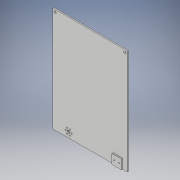
# Autodesk Inventor part: ElectronicsPlate
Saved by Autodesk Inventor 2017 (Build 210142000, 142)
## iProperties
Created: 2018-01-06
Part Number: ElectronicsPlate
Material: Generic
Document SubType Name: Modeling
Designer: User
Density: 1 g/cm^3
Appearance: Default
Author: User
Autodesk Inventor part; units mm, degrees
ref_plane "YZ Plane" through (0, 0, 0) normal (1, 0, 0) x (0, 1, 0)
ref_plane "XZ Plane" through (0, 0, 0) normal (0, 1, 0) x (-1, 0, 0)
ref_plane "XY Plane" through (0, 0, 0) normal (0, 0, 1) x (1, 0, 0)
sketch "Sketch1" plane through (0, 0, 0) normal (0, 0, 1) x (1, 0, 0)
  line L0 (0, 0) -> (199.39, 0)
  line L1 (199.39, 0) -> (199.39, 266.7)
  line L2 (199.39, 266.7) -> (0, 266.7)
  line L3 (0, 266.7) -> (0, 0)
  line L4 (12.1493, 266.7) -> (12.1493, 263.525)
  line L5 (0, 247.1772) -> (3.175, 247.1772)
  line L6 (3.175, 263.525) -> (147.2946, 263.525)
  line L7 (147.2946, 263.525) -> (147.2946, 161.925)
  line L8 (147.2946, 161.925) -> (3.175, 161.925)
  line L9 (3.175, 161.925) -> (3.175, 263.525)
  line L10 (5.8968, 161.925) -> (5.8968, 158.75)
  line L11 (3.175, 158.75) -> (147.2946, 158.75)
  line L12 (147.2946, 158.75) -> (147.2946, 57.15)
  line L13 (147.2946, 57.15) -> (3.175, 57.15)
  line L14 (3.175, 57.15) -> (3.175, 158.75)
  line L15 (147.2946, 247.6224) -> (150.4696, 247.6224)
  line L16 (150.4696, 199.39) -> (186.0296, 199.39)
  line L17 (186.0296, 199.39) -> (186.0296, 107.95)
  line L18 (186.0296, 107.95) -> (150.4696, 107.95)
  line L19 (150.4696, 107.95) -> (150.4696, 199.39)
  dimension "d0" = 199.39
  dimension "d2" = 3.175
  dimension "d3" = 3.175
  dimension "d4" = 144.1196
  dimension "d5" = 101.6
  dimension "d6" = 3.175
  dimension "d7" = 101.6
  dimension "d8" = 3.175
  dimension "d9" = 35.56
  dimension "d10" = 91.44
  dimension "d11" = 107.95
  dimension "d12" = 3.175
  dimension "d13" = 3.175
  constraints: 40 end point, 8 parallel, 7 perpendicular, 5 horizontal, 4 point on line
  measures "d0" distance of L2.end L1.end
  measures "d2" distance of L4.start L4.end
  measures "d3" distance of L5.start L5.end
  measures "d4" distance of L7.end L8.end
  measures "d5" distance of L6.end L7.end
  measures "d6" distance of L10.start L10.end
  measures "d7" distance of L11.end L12.end
  measures "d8" distance of L15.start L15.end
  measures "d9" distance of L17.end L18.end
  measures "d10" distance of L16.end L17.end
  measures "d11" distance between parallel lines of L0 L18
  measures "d12" distance between parallel lines of L2 L6
  measures "d13" distance between parallel lines of L8 L11
sketch "Sketch2" plane through (0, 0, 0) normal (0, 0, 1) x (1, 0, 0)
  line L0 (199.39, 0) -> (0, 0)
  line L1 (0, 0) -> (0, 266.7)
  line L2 (0, 266.7) -> (199.39, 266.7)
  line L3 (199.39, 266.7) -> (199.39, 0)
  point P0 (0, 0)
  constraints: 8 end point, 2 parallel, 1 horizontal, 1 perpendicular
extrude "Extrusion1" add sketch "Sketch2" along normal blind 3.175
sketch "Sketch3" plane through (0, 0, 3.175) normal (0, 0, 1) x (1, 0, 0)
  line L0 (33.6942, 0) -> (33.6942, 14.605)
  line L1 (0, 14.605) -> (42.5196, 14.605)
  line L2 (0, 14.605) -> (42.5196, 14.605) construction
  circle A0 centre (42.5196, 14.605) radius 8.001
  circle A1 centre (42.5196, 14.605) radius 3.4925
  circle A2 centre (34.5186, 14.605) radius 1.5875
  circle A3 centre (38.5191, 7.6759) radius 1.5875
  circle A4 centre (46.5201, 7.6759) radius 1.5875
  circle A5 centre (50.5206, 14.605) radius 1.5875
  circle A6 centre (46.5201, 21.5341) radius 1.5875
  circle A7 centre (38.5191, 21.5341) radius 1.5875
  dimension "d20" = 16.002
  dimension "d16" = 14.605
  dimension "d18" = 42.5196
  dimension "d19" = 0
  dimension "d21" = 6.985
  dimension "d22" = 3.175
  dimension "d27" = 360
  constraints: 7 centre point, 6 end point, 2 coincident, 1 collinear, 1 horizontal, 1 horizontal alignment, 1 point on line, 15 other
  measures "d16" distance of L0.start L0.end
  measures "d18" distance of L1.start L1.end
  measures "d19" distance between parallel lines of L1 L2
  measures "d21" diameter of A1
  measures "d22" diameter of A2
extrude "Extrusion2" cut sketch "Sketch3" against normal blind 6.35 contours A2 L1 L0 | L0 L1 A0 A2 | L1 A2 A0 | A0 L1 A2 | A0 A2 L1 | A3 A0 | A0 A3 | A7 A0 | A0 A7 | A4 A0 | A0 A4 | A6 A0 | A0 A6 | A5 A0 | A0 A5 | A1
sketch "Sketch4" plane through (0, 0, 0) normal (0, 0, -1) x (-1, 0, 0)
  line L0 (-199.39, 0) -> (-199.39, 266.7) projected
  line L1 (-199.39, 15.2095) -> (-180.34, 15.2095)
  line L2 (-199.39, 15.2095) -> (-180.34, 15.2095) construction
  line L3 (0, 0) -> (-199.39, 0) projected
  line L4 (-180.34, 0) -> (-180.34, 12.7)
  line L5 (-180.34, 0) -> (-167.64, 0) construction
  line L6 (-180.34, 12.7) -> (-167.64, 12.7)
  circle A0 centre (-180.34, 12.7) radius 1.7526
  circle A1 centre (-167.64, 12.7) radius 1.7526
  dimension "d29" = 19.05
  dimension "d30" = 0
  dimension "d31" = 12.7
  dimension "d32" = 90
  dimension "d33" = 12.7
  dimension "d34" = 3.5052
  dimension "d35" = 3.5052
  dimension "d48" = 0
  constraints: 10 end point, 3 horizontal, 2 centre point, 2 coincident, 2 equal length, 2 perpendicular, 2 point on line
  measures "d29" distance of L1.start L1.end
  measures "d30" distance between parallel lines of L1 L2
  measures "d31" distance of L4.start L4.end
  measures "d32" angle of L5 L4
  measures "d33" distance of L4.end L6.end
  measures "d34" diameter of A0
  measures "d35" diameter of A1
  measures "d48" distance from line of L1.end L4
hole "Hole1" at (180.34, 12.7, 0) at (167.64, 12.7, 0) direction (0, 0, 1) diameter 2.6416 depth 10.9728 tip angle 118 thread size "6-32 UNC" class "2B" standard "ANSI Unified Screw Threads"
sketch "Sketch5" plane through (0, 0, 3.175) normal (0, 0, 1) x (1, 0, 0)
  circle A0 centre (180.34, 12.7) radius 1.3208 projected
  line L0 (180.34, 12.7) -> (186.69, 12.7)
  circle A1 centre (167.64, 12.7) radius 1.3208 projected
  line L1 (167.64, 12.7) -> (161.29, 12.7)
  line L2 (0, 0) -> (199.39, 0) projected
  line L3 (186.69, 0) -> (161.29, 0)
  line L4 (161.29, 0) -> (161.29, 25.4)
  line L5 (161.29, 25.4) -> (186.69, 25.4)
  line L6 (186.69, 25.4) -> (186.69, 0)
  dimension "d43" = 6.35
  dimension "d44" = 6.35
  dimension "d45" = 25.4
  constraints: 12 end point, 3 horizontal, 2 parallel, 1 perpendicular, 1 point on line
  measures "d43" distance of L0.start L0.end
  measures "d44" distance of L1.start L1.end
  measures "d45" distance of L3.end L4.end
extrude "Extrusion3" add sketch "Sketch5" along normal blind 3.175
sketch "Sketch6" plane through (0, 0, 3.175) normal (0, 0, 1) x (1, 0, 0)
  point P0 (0, 0)
sketch "Sketch7" plane through (0, 0, 3.175) normal (0, 0, 1) x (1, 0, 0)
  line L0 (199.39, 266.7) -> (0, 266.7) projected
  line L1 (0, 266.7) -> (199.39, 266.7)
  line L2 (199.39, 266.7) -> (199.39, 279.4)
  line L3 (199.39, 279.4) -> (0, 279.4)
  line L4 (0, 279.4) -> (0, 266.7)
  line L5 (199.39, 0) -> (199.39, 266.7) projected
  point P0 (0, 0)
  dimension "d49" = 12.7
  dimension "d50" = 0
  constraints: 8 end point, 2 parallel, 1 horizontal, 1 perpendicular
  measures "d49" distance of L2.end L1.end
  measures "d50" distance between parallel lines of L2 L5
extrude "Extrusion4" add sketch "Sketch7" against normal blind 3.175
sketch "Sketch9" plane through (0, 0, 3.175) normal (0, 0, 1) x (1, 0, 0)
  line L0 (199.39, 279.4) -> (0, 279.4) projected
  line L1 (0, 279.4) -> (6.35, 279.4)
  line L2 (6.35, 279.4) -> (6.35, 273.05)
  line L3 (6.35, 273.05) -> (0, 273.05)
  line L4 (0, 273.05) -> (0, 279.4)
  line L5 (199.39, 0) -> (199.39, 279.4) projected
  line L6 (199.39, 279.4) -> (193.04, 279.4)
  line L7 (193.04, 279.4) -> (193.04, 273.05)
  line L8 (193.04, 273.05) -> (199.39, 273.05)
  line L9 (199.39, 273.05) -> (199.39, 279.4)
  point P0 (0, 0)
  dimension "d64" = 6.35
  dimension "d65" = 6.35
  dimension "d66" = 6.35
  dimension "d67" = 6.35
  constraints: 16 end point, 4 parallel, 2 coincident, 2 horizontal, 2 perpendicular
  measures "d64" distance of L2.end L3.end
  measures "d65" distance of L1.end L2.end
  measures "d66" distance of L8.end L7.end
  measures "d67" distance of L7.end L6.end
hole "Hole3" at (6.35, 273.05, 3.175) at (193.04, 273.05, 3.175) direction (0, 0, -1) diameter 6.35 depth 9.525 tip angle 118
body "Solid1"
